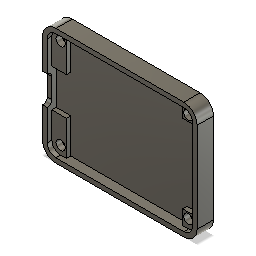
Icebreaker Case Bottom (Autodesk Fusion 360 design; units mm, degrees)
Autodesk Fusion 360 part; units mm, degrees
sketch "Sketch1" plane through (0, 0, 0) normal (0, 0, 1) x (1, 0, 0)
  line L0 (0, 0) -> (53.2, 0)
  line L1 (53.2, 0) -> (53.2, 40.2)
  line L2 (53.2, 40.2) -> (0, 40.2)
  line L3 (0, 40.2) -> (0, 0)
  circle A0 centre (4.6, 35.6) radius 1.6
  circle A1 centre (4.6, 4.6) radius 1.6
  circle A2 centre (48.6, 35.6) radius 1.6
  circle A3 centre (48.6, 4.6) radius 1.6
  dimension "d1" = 53.2
  dimension "d2" = 40.2
  dimension "d3" = 3.2
  dimension "d4" = 3.2
  dimension "d5" = 3.2
  dimension "d6" = 3.2
  dimension "d7" = 4.6
  dimension "d8" = 4.6
  dimension "d9" = 4.6
  dimension "d10" = 4.6
  dimension "d11" = 4.6
  dimension "d12" = 4.6
  dimension "d13" = 4.6
  dimension "d14" = 4.6
  measures "d1" distance of L0.start
  measures "d2" distance of L0.start
  measures "d3" diameter of A0
  measures "d4" diameter of A1
  measures "d5" diameter of A2
  measures "d6" diameter of A3
  measures "d7" distance of L3
  measures "d8" distance of L2
  measures "d10" distance of L0.start
  measures "d11" distance of L0.start
  measures "d13" distance of L2 L0.start
extrude "Extrude1" add sketch "Sketch1" along normal blind 4
sketch "Sketch2" plane through (0, 0, 0) normal (0, 0, -1) x (-1, 0, 0)
  circle A0 centre (-48.6, 4.6) radius 1.6
  circle A1 centre (-4.6, 4.6) radius 1.6
  circle A2 centre (-48.6, 35.6) radius 1.6
  circle A3 centre (-4.6, 35.6) radius 1.6
  line L0 (0, 0) -> (0, 40.2)
  line L1 (0, 40.2) -> (-53.2, 40.2)
  line L2 (-53.2, 40.2) -> (-53.2, 0)
  line L3 (-53.2, 0) -> (0, 0)
  line L4 (-3.0123, 32.85) -> (-1.4246, 35.6)
  line L5 (-1.4246, 35.6) -> (-3.0123, 38.35)
  line L6 (-3.0123, 38.35) -> (-6.1877, 38.35)
  line L7 (-6.1877, 38.35) -> (-7.7754, 35.6)
  line L8 (-7.7754, 35.6) -> (-6.1877, 32.85)
  line L9 (-6.1877, 32.85) -> (-3.0123, 32.85)
  line L10 (-47.0123, 32.85) -> (-45.4246, 35.6)
  line L11 (-45.4246, 35.6) -> (-47.0123, 38.35)
  line L12 (-47.0123, 38.35) -> (-50.1877, 38.35)
  line L13 (-50.1877, 38.35) -> (-51.7754, 35.6)
  line L14 (-51.7754, 35.6) -> (-50.1877, 32.85)
  line L15 (-50.1877, 32.85) -> (-47.0123, 32.85)
  line L16 (-50.1877, 7.35) -> (-51.7754, 4.6)
  line L17 (-51.7754, 4.6) -> (-50.1877, 1.85)
  line L18 (-50.1877, 1.85) -> (-47.0123, 1.85)
  line L19 (-47.0123, 1.85) -> (-45.4246, 4.6)
  line L20 (-45.4246, 4.6) -> (-47.0123, 7.35)
  line L21 (-47.0123, 7.35) -> (-50.1877, 7.35)
  line L22 (-6.1877, 7.35) -> (-7.7754, 4.6)
  line L23 (-7.7754, 4.6) -> (-6.1877, 1.85)
  line L24 (-6.1877, 1.85) -> (-3.0123, 1.85)
  line L25 (-3.0123, 1.85) -> (-1.4246, 4.6)
  line L26 (-1.4246, 4.6) -> (-3.0123, 7.35)
  line L27 (-3.0123, 7.35) -> (-6.1877, 7.35)
  dimension "d17" = 2.75
  dimension "d18" = 2.75
  dimension "d19" = 2.75
  dimension "d20" = 2.75
  measures "d17" distance of L9
  measures "d18" distance of L21
  measures "d20" distance of L27
extrude "Extrude2" cut sketch "Sketch2" against normal blind 2 contours L4 L5 L6 L7 L8 L9 | L10 L11 L12 L13 L14 L15 | L16 L17 L18 L19 L20 L21 | L22 L23 L24 L25 L26 L27
fillet "Fillet1" radius 4.6 4 edges at (53.2, 40.2, 2) (53.2, 0, 2) (0, 0, 2) (0, 40.2, 2)
sketch "Sketch4" plane through (0, 0, 4) normal (0, 0, 1) x (1, 0, 0)
  arc A0 (4.6, 40.2) -> (0, 35.6) centre (4.6, 35.6) ccw
  line L0 (0, 35.6) -> (0, 4.6)
  arc A1 (0, 4.6) -> (4.6, 0) centre (4.6, 4.6) ccw
  line L1 (4.6, 0) -> (48.6, 0)
  arc A2 (48.6, 0) -> (53.2, 4.6) centre (48.6, 4.6) ccw
  line L2 (53.2, 4.6) -> (53.2, 35.6)
  arc A3 (53.2, 35.6) -> (48.6, 40.2) centre (48.6, 35.6) ccw
  line L3 (48.6, 40.2) -> (4.6, 40.2)
  circle A4 centre (4.6, 4.6) radius 1.6
  circle A5 centre (48.6, 35.6) radius 1.6
  circle A6 centre (4.6, 35.6) radius 1.6
  circle A7 centre (48.6, 4.6) radius 1.6
  line L4 (1.6, 35.6) -> (1.6, 4.6)
  arc A8 (1.6, 4.6) -> (4.6, 1.6) centre (4.6, 4.6) ccw
  line L5 (4.6, 1.6) -> (48.6, 1.6)
  arc A9 (48.6, 1.6) -> (51.6, 4.6) centre (48.6, 4.6) ccw
  line L6 (51.6, 4.6) -> (51.6, 35.6)
  arc A10 (51.6, 35.6) -> (48.6, 38.6) centre (48.6, 35.6) ccw
  line L7 (48.6, 38.6) -> (4.6, 38.6)
  arc A11 (4.6, 38.6) -> (1.6, 35.6) centre (4.6, 35.6) ccw
  dimension "d24" = 1.6
  measures "d24" distance of L0
extrude "Extrude3" add sketch "Sketch4" along normal blind 1.6 contours A0 L0 A1 L1 A2 L2 A3 L3
sketch "Sketch5" plane through (0, 0, 4) normal (0, 0, 1) x (1, 0, 0)
  line L0 (1.6, 35.6) -> (1.6, 4.6)
  arc A0 (1.6, 4.6) -> (4.6, 1.6) centre (4.6, 4.6) ccw
  line L1 (4.6, 1.6) -> (48.6, 1.6)
  arc A1 (48.6, 1.6) -> (51.6, 4.6) centre (48.6, 4.6) ccw
  line L2 (51.6, 4.6) -> (51.6, 35.6)
  arc A2 (51.6, 35.6) -> (48.6, 38.6) centre (48.6, 35.6) ccw
  line L3 (48.6, 38.6) -> (4.6, 38.6)
  arc A3 (4.6, 38.6) -> (1.6, 35.6) centre (4.6, 35.6) ccw
  circle A4 centre (4.6, 4.6) radius 1.6
  circle A5 centre (48.6, 35.6) radius 1.6
  circle A6 centre (4.6, 35.6) radius 1.6
  circle A7 centre (48.6, 4.6) radius 1.6
  line L4 (1.6, 13.6) -> (6.6, 13.6)
  line L5 (6.6, 13.6) -> (6.6, 1.6)
  line L6 (46.6, 1.6) -> (46.6, 6.6)
  line L7 (46.6, 6.6) -> (51.6, 6.6)
  line L8 (1.6, 26.6) -> (6.6, 26.6)
  line L9 (6.6, 26.6) -> (6.6, 38.6)
  line L10 (46.6, 38.6) -> (46.6, 33.6)
  line L11 (46.6, 33.6) -> (51.6, 33.6)
  dimension "d27" = 12
  dimension "d28" = 5
  dimension "d29" = 5
  dimension "d30" = 12
  dimension "d31" = 5
  dimension "d32" = 5
  dimension "d33" = 5
  dimension "d34" = 5
extrude "Extrude4" cut sketch "Sketch5" against normal blind 1.5 contours L0 L1 L2 L3 L4 L5 L6 L7 L8 L9 L10 L11
sketch "Sketch6" plane through (0, 0, 5.6) normal (0, 0, 1) x (1, 0, 0)
  arc A0 (4.6, 38.6) -> (1.6, 35.6) centre (4.6, 35.6) ccw
  line L0 (4.6, 38.6) -> (48.6, 38.6)
  arc A1 (51.6, 35.6) -> (48.6, 38.6) centre (48.6, 35.6) ccw
  line L1 (51.6, 35.6) -> (51.6, 4.6)
  arc A2 (48.6, 1.6) -> (51.6, 4.6) centre (48.6, 4.6) ccw
  line L2 (48.6, 1.6) -> (4.6, 1.6)
  arc A3 (1.6, 4.6) -> (4.6, 1.6) centre (4.6, 4.6) ccw
  line L3 (1.6, 4.6) -> (1.6, 35.6)
  line L4 (48.6, 40.2) -> (4.6, 40.2)
  arc A4 (4.6, 40.2) -> (0, 35.6) centre (4.6, 35.6) ccw
  line L5 (0, 35.6) -> (0, 4.6)
  arc A5 (0, 4.6) -> (4.6, 0) centre (4.6, 4.6) ccw
  line L6 (4.6, 0) -> (48.6, 0)
  arc A6 (48.6, 0) -> (53.2, 4.6) centre (48.6, 4.6) ccw
  line L7 (53.2, 4.6) -> (53.2, 35.6)
  arc A7 (53.2, 35.6) -> (48.6, 40.2) centre (48.6, 35.6) ccw
  line L8 (0, 25.1) -> (1.6, 25.1)
  line L9 (0, 15.1) -> (1.6, 15.1)
  dimension "d37" = 10
  dimension "d38" = 10.5
  measures "d37" distance of L8 L9
  measures "d38" distance of L9
extrude "Extrude5" cut sketch "Sketch6" against normal blind 1.6 contours L3 L5 L8 L9
fillet "Fillet2" radius 1.6 2 edges at (0.8, 25.1, 4) (0.8, 15.1, 4)
equation "d1 = 50 mm + ( ( 2 * 1.6 ) * 1 mm )"
equation "d2 = 37 mm + ( ( 2 * 1.6 ) * 1 mm )"
equation "d7 = 3 mm + 1.6 mm"
equation "d8 = d7"
equation "d9 = d7"
equation "d10 = d7"
equation "d11 = d7"
equation "d12 = d7"
equation "d13 = d7"
equation "d14 = d7"
equation "d17 = ( 5.5 / 2 ) * 1 mm"
equation "d18 = d17"
equation "d19 = d17"
equation "d20 = d17"
equation "d23 = 3 mm + 1.6 mm"
equation "d29 = d28"
equation "d30 = d27"
